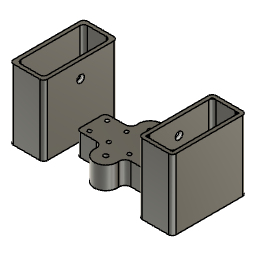
Camera Tilt Mount (Autodesk Fusion 360 design; units mm, degrees)
Autodesk Fusion 360 part; units mm, degrees
sketch "Sketch1" plane through (0, 0, 0) normal (0, 0, 1) x (1, 0, 0)
  circle A0 centre (0, 0) radius 11.25
  line L0 (0, 0) -> (0, 15)
  line L1 (0, 15) -> (0, -15)
  circle A1 centre (0, 15) radius 1.5
  circle A2 centre (0, -15) radius 1.5
  line L2 (0, 0) -> (7.955, -7.955)
  line L3 (0, 0) -> (11.25, 0) construction
  line L4 (0, 0) -> (-7.955, -7.955)
  line L5 (-7.955, -7.955) -> (7.955, -7.955)
  line L6 (-7.955, -7.955) -> (7.955, -7.955)
  line L7 (-7.955, -7.955) -> (-7.955, 7.955)
  line L8 (-7.955, 7.955) -> (7.955, 7.955)
  line L9 (-7.955, 7.955) -> (7.955, 7.955)
  line L10 (0, 0) -> (32.5, 0)
  line L11 (32.5, 0) -> (0, 0)
  line L12 (0, 0) -> (-32.5, 0)
  line L13 (32.5, 0) -> (4.5, 0)
  line L14 (-32.5, 0) -> (-4.5, 0)
  line L15 (-4.5, 0) -> (-22.5, 0)
  line L16 (0, 0) -> (18, 0)
  line L17 (32.5, 0) -> (22.5, 0)
  line L18 (4.5, 0) -> (4.5, 22.5)
  line L19 (4.5, 22.5) -> (22.5, 22.5)
  line L20 (22.5, 22.5) -> (22.5, -22.5)
  line L21 (22.5, -22.5) -> (4.5, -22.5)
  line L22 (4.5, -22.5) -> (4.5, 0)
  line L23 (4.5, 22.5) -> (2, 22.5)
  line L24 (2, 22.5) -> (2, 25)
  line L25 (2, 22.5) -> (2, -25)
  line L26 (2, -25) -> (25, -25)
  line L27 (25, -25) -> (25, 25)
  line L28 (25, 25) -> (2, 25)
  circle A3 centre (0, 15) radius 7.75
  circle A4 centre (0, -15) radius 7.75
  line L29 (-32.5, 0) -> (-4.5, 0)
  line L30 (-4.5, 0) -> (-4.5, 22.5)
  line L31 (-4.5, 22.5) -> (-4.5, -22.5)
  line L32 (-4.5, -22.5) -> (-22.5, -22.5)
  line L33 (-22.5, -22.5) -> (-22.5, 22.5)
  line L34 (-22.5, 22.5) -> (-4.5, 22.5)
  line L35 (-4.5, 22.5) -> (-4.5, 25)
  line L36 (-4.5, 25) -> (-2, 25)
  line L37 (-2, 25) -> (-2, -25)
  line L38 (-2, -25) -> (-25, -25)
  line L39 (-25, -25) -> (-25, 25)
  line L40 (-25, 25) -> (-4.5, 25)
  dimension "d1" = 22.5
  dimension "d2" = 15
  dimension "d3" = 30
  dimension "d4" = 3
  dimension "d5" = 3
  dimension "d6" = 45
  dimension "d7" = 90
  dimension "d10" = 32.5
  dimension "d11" = 32.5
  dimension "d12" = 28
  dimension "d13" = 28
  dimension "d14" = 18
  dimension "d15" = 18
  dimension "d18" = 10
  dimension "d19" = 22.5
  dimension "d20" = 18
  dimension "d21" = 45
  dimension "d22" = 47.5
  dimension "d23" = 23
  dimension "d24" = 15.5
  dimension "d25" = 15.5
  dimension "d26" = 28
  dimension "d27" = 22.5
  dimension "d28" = 45
  dimension "d29" = 18
  constraint coincident A0.centre L0.start
  constraint vertical L0
  constraint parallel L0 L1
  constraint coincident L0.end L1.start
  constraint coincident L1.end A2.centre
  constraint horizontal L3
  constraint coincident A0 L2.end
  constraint coincident A0 L4.end
  constraint horizontal L6
  constraint coincident A0 L7.end
  constraint perpendicular L5 L7
  constraint coincident A0 L8.end
  constraint perpendicular L7 L8
  constraint horizontal L9
  constraint perpendicular L1 L10
  constraint perpendicular L0 L12
  constraint parallel L10 L13
  constraint perpendicular L7 L14
  constraint parallel L12 L15
  constraint parallel L10 L16
  constraint parallel L11 L17
  constraint perpendicular L13 L18
  constraint perpendicular L18 L19
  constraint perpendicular L19 L20
  constraint perpendicular L20 L21
  constraint perpendicular L11 L22
  constraint perpendicular L18 L23
  constraint perpendicular L23 L24
  constraint perpendicular L23 L25
  constraint perpendicular L25 L26
  constraint perpendicular L26 L27
  constraint perpendicular L24 L28
  constraint concentric A1 A3
  constraint concentric A2 A4
  constraint parallel L14 L29
  constraint perpendicular L14 L30
  constraint parallel L30 L31
  constraint perpendicular L31 L32
  constraint perpendicular L32 L33
  constraint perpendicular L30 L34
  constraint perpendicular L34 L35
  constraint perpendicular L35 L36
  constraint perpendicular L36 L37
  constraint perpendicular L37 L38
  constraint perpendicular L38 L39
  constraint perpendicular L35 L40
  measures "d1" diameter of A0
  measures "d2" distance of A0.centre L0.end
  measures "d3" distance of L0.end L1.end
  measures "d4" diameter of A1
  measures "d5" diameter of A2
  measures "d6" angle of L2 L3
  measures "d7" angle of L2 L4
  measures "d10" distance of A0.centre L10.end
  measures "d11" distance of A0.centre L12.end
  measures "d12" distance of L10.end L13.end
  measures "d13" distance of L12.end L14.end
  measures "d14" distance of L14.end L15.end
  measures "d15" distance of A0.centre L16.end
  measures "d18" distance of L10.end L17.end
  measures "d19" distance of L13.end L18.end
  measures "d20" distance of L18.end L19.end
  measures "d21" distance of L19.end L20.end
  measures "d22" distance of L23.end L25.end
  measures "d23" distance of L25.end L26.end
  measures "d24" diameter of A3
  measures "d25" diameter of A4
  measures "d26" distance of L12.end L14.end
  measures "d27" distance of L14.end L30.end
  measures "d28" distance of L30.end L31.end
  measures "d29" distance of L31.end L32.end
extrude "Extrude1" add sketch "Sketch1" along normal blind 50 contours L2 L10 L11 L16 L22 L25 | L8 L9 L10 L11 L16 L18 L25 A3 | L8 L9 L18 A3 | L2 L5 L6 L22 L25 A4 | L5 L6 L22 A4 | L10 L11 L13 L17 L19 L20 L23 L24 L27 L28 | L10 L11 L13 L17 L20 L21 L22 L25 L26 L27 A4 | A0 L8 L9 L18 L25 A3 | A0 L18 L25 A3 | L8 L9 L25 A3 | A0 L22 L25 A4 | A0 L5 L6 L22 L25 A4 | L5 L6 L25 A4 | L18 L23 L25 A3 | L4 L5 L6 A4 L31 L37 | L4 L12 L31 L37 | L8 L9 L12 A3 L30 L31 L37 | L8 L9 A3 L37 | L5 L6 A4 L37 | A0 L8 L9 A3 L30 L31 L37 | A0 A3 L30 L31 L37 | A3 L30 L31 L35 L36 L37 | A0 A4 L31 L37 | A0 L5 L6 A4 L31 L37 | L12 L14 A4 L29 L31 L32 L33 L37 L38 L39 | L8 L9 A3 L30 L31 | L5 L6 A4 L31 | L12 L14 L29 L33 L34 L35 L39 L40 makes body 1 at (-2, 8.3333, 16.6667) makes body 2 at (2, 8.3333, 16.6667)
extrude "Extrude2" add sketch "Sketch1" along normal blind 2.5 separate body contours A0 L8 L9 L10 L11 L13 L16 L18 | A0 L10 L11 L13 L16 L20 L21 L22 A4 | A0 L2 L10 L11 L13 L16 L22 | A0 L10 L11 L13 L16 L18 L19 L20 A3 | A0 L8 L9 L18 A3 | L2 L5 L6 L22 | A0 L5 L6 L22 A4 | A0 L18 A3 | A0 L18 A3 | A0 L22 A4 | A0 L22 A4 | L4 L5 L6 L31 | L4 L7 L12 L14 L15 L29 L31 | L7 L8 L9 L12 L14 L15 L29 L30 L31 | A0 L12 L14 L15 A4 L29 L31 L32 L33 | A0 L5 L6 A4 L31 | A0 L7 L12 L14 L15 L29 | A0 L7 L12 L14 L15 L29 | A0 L8 L9 A3 L30 L31 | A0 A3 L30 L31 | A0 A3 L30 L31 | A0 L12 L14 L15 A3 L29 L30 L31 L33 L34 | A0 A4 L31 | A0 A4 L31 makes body 3 at (-10.5, -7.5, 0) makes body 4 at (16.5, -7.5, 0)
extrude "Extrude4" add sketch "Sketch1" against normal blind 10 separate body contours A0 L8 L9 L10 L11 L13 L16 L18 | A0 L2 L10 L11 L13 L16 L22 | A0 L8 L9 L18 A3 | L2 L5 L6 L22 | A0 L5 L6 L22 A4 | L2 L10 L11 L16 L22 L25 | L8 L9 L10 L11 L16 L18 L25 A3 | A0 L18 A3 | A0 L18 A3 | L8 L9 L18 A3 | A0 L22 A4 | A0 L22 A4 | L2 L5 L6 L22 L25 A4 | L5 L6 L22 A4 | L2 L10 L11 L16 L25 | L0 L1 L10 L11 L16 L25 A3 | A0 L8 L9 L18 L25 A3 | A0 L18 L25 A3 | L8 L9 L25 A3 | A0 L22 L25 A4 | A0 L5 L6 L22 L25 A4 | L1 L2 L25 A4 | L5 L6 L25 A4 | L0 L1 L12 A3 L37 | L1 L4 A4 L37 | L4 L12 L37 | L0 L1 L8 L9 L25 A3 | A0 L0 L1 L8 L9 L25 | A0 L25 A3 L37 | A0 L25 A4 L37 | A0 L1 L5 L6 L25 | L1 L5 L6 L25 A4 | L0 L1 L8 L9 A3 L37 | L1 L5 L6 A4 L37 | L4 L5 L6 A4 L31 L37 | L4 L12 L31 L37 | L8 L9 L12 A3 L30 L31 L37 | A0 L0 L1 L8 L9 L37 | A0 L1 L5 L6 L37 | L8 L9 A3 L37 | L5 L6 A4 L37 | L4 L5 L6 L31 | L4 L7 L12 L14 L15 L29 L31 | L7 L8 L9 L12 L14 L15 L29 L30 L31 | A0 L8 L9 A3 L30 L31 L37 | A0 A3 L30 L31 L37 | A0 A4 L31 L37 | A0 L5 L6 A4 L31 L37 | L8 L9 A3 L30 L31 | L5 L6 A4 L31 | A0 L5 L6 A4 L31 | A0 L7 L12 L14 L15 L29 | A0 L7 L12 L14 L15 L29 | A0 L8 L9 A3 L30 L31 | A0 A3 L30 L31 | A0 A3 L30 L31 | A0 A4 L31 | A0 A4 L31 makes body 5
extrude "Extrude5" add sketch "Sketch1" along normal blind 2.5 contours A0 L8 L9 L10 L11 L13 L16 L18 | A0 L10 L11 L13 L16 L20 L21 L22 A4 | A0 L2 L10 L11 L13 L16 L22 | A0 L10 L11 L13 L16 L18 L19 L20 A3 | A0 L8 L9 L18 A3 | L2 L5 L6 L22 | A0 L5 L6 L22 A4 | A0 L18 A3 | A0 L18 A3 | A0 L22 A4 | A0 L22 A4 | L4 L5 L6 L31 | L4 L7 L12 L14 L15 L29 L31 | L7 L8 L9 L12 L14 L15 L29 L30 L31 | A0 L12 L14 L15 A4 L29 L31 L32 L33 | A0 L5 L6 A4 L31 | A0 L7 L12 L14 L15 L29 | A0 L7 L12 L14 L15 L29 | A0 L8 L9 A3 L30 L31 | A0 A3 L30 L31 | A0 A3 L30 L31 | A0 L12 L14 L15 A3 L29 L30 L31 L33 L34 | A0 A4 L31 | A0 A4 L31 bodies 5
extrude "Extrude6" cut sketch "Sketch1" along normal blind 1 contours A0 L8 L9 L10 L11 L13 L16 L18 | A0 L10 L11 L13 L16 L20 L21 L22 A4 | A0 L2 L10 L11 L13 L16 L22 | A0 L10 L11 L13 L16 L18 L19 L20 A3 | A0 L8 L9 L18 A3 | L2 L5 L6 L22 | A0 L5 L6 L22 A4 | A0 L18 A3 | A0 L18 A3 | A0 L22 A4 | A0 L22 A4 | L4 L5 L6 L31 | L4 L7 L12 L14 L15 L29 L31 | L7 L8 L9 L12 L14 L15 L29 L30 L31 | A0 L12 L14 L15 A4 L29 L31 L32 L33 | A0 L5 L6 A4 L31 | A0 L7 L12 L14 L15 L29 | A0 L7 L12 L14 L15 L29 | A0 L8 L9 A3 L30 L31 | A0 A3 L30 L31 | A0 A3 L30 L31 | A0 L12 L14 L15 A3 L29 L30 L31 L33 L34 | A0 A4 L31 | A0 A4 L31 bodies 5 makes body 6 at (-10.5, -7.5, 1) makes body 7 at (2.8306, -3.9262, -10)
extrude "Extrude7" add sketch "Sketch1" along normal blind 50 contours L2 L10 L11 L16 L22 L25 | L8 L9 L10 L11 L16 L18 L25 A3 | L8 L9 L18 A3 | L2 L5 L6 L22 L25 A4 | L5 L6 L22 A4 | L10 L11 L13 L17 L19 L20 L23 L24 L27 L28 | L10 L11 L13 L17 L20 L21 L22 L25 L26 L27 A4 | A0 L8 L9 L18 L25 A3 | A0 L18 L25 A3 | L8 L9 L25 A3 | A0 L22 L25 A4 | A0 L5 L6 L22 L25 A4 | L5 L6 L25 A4 | L18 L23 L25 A3 | L4 L5 L6 A4 L31 L37 | L4 L12 L31 L37 | L8 L9 L12 A3 L30 L31 L37 | L8 L9 A3 L37 | L5 L6 A4 L37 | A0 L8 L9 A3 L30 L31 L37 | A0 A3 L30 L31 L37 | A3 L30 L31 L35 L36 L37 | A0 A4 L31 L37 | A0 L5 L6 A4 L31 L37 | L12 L14 A4 L29 L31 L32 L33 L37 L38 L39 | L8 L9 A3 L30 L31 | L5 L6 A4 L31 | L12 L14 L29 L33 L34 L35 L39 L40 bodies 5 6 7
extrude "Extrude8" cut sketch "Sketch1" along normal blind 1 contours L2 L10 L11 L16 L22 L25 | L8 L9 L10 L11 L16 L18 L25 A3 | L8 L9 L18 A3 | L2 L5 L6 L22 L25 A4 | L5 L6 L22 A4 | L10 L11 L13 L17 L19 L20 L23 L24 L27 L28 | L10 L11 L13 L17 L20 L21 L22 L25 L26 L27 A4 | A0 L8 L9 L18 L25 A3 | A0 L18 L25 A3 | L8 L9 L25 A3 | A0 L22 L25 A4 | A0 L5 L6 L22 L25 A4 | L5 L6 L25 A4 | L18 L23 L25 A3 | L4 L5 L6 A4 L31 L37 | L4 L12 L31 L37 | L8 L9 L12 A3 L30 L31 L37 | L8 L9 A3 L37 | L5 L6 A4 L37 | A0 L8 L9 A3 L30 L31 L37 | A0 A3 L30 L31 L37 | A3 L30 L31 L35 L36 L37 | A0 A4 L31 L37 | A0 L5 L6 A4 L31 L37 | L12 L14 A4 L29 L31 L32 L33 L37 L38 L39 | L8 L9 A3 L30 L31 | L5 L6 A4 L31 | L12 L14 L29 L33 L34 L35 L39 L40 bodies 5 makes body 8 at (2, 8.3333, 17.3333) makes body 9 at (-2, 8.3333, 17.3333)
extrude "Extrude9" add 2 faces at (24.1667, 7.5, 50) (-24.1667, 7.5, 50) along direction (0, 0, 1) blind 1 on bodies 8 9 bodies 8 9
sketch "Sketch2" plane through (0, 0, -10) normal (0, 0, -1) x (1, 0, 0)
  circle A0 centre (0, 15) radius 1.5
  circle A1 centre (0, -15) radius 1.5
  arc A2 (5.67, 9.7167) -> (-5.67, 9.7167) centre (0, 15) ccw
  arc A3 (-5.67, 9.7167) -> (-5.67, -9.7167) centre (0, 0) ccw
  arc A4 (-5.67, -9.7167) -> (5.67, -9.7167) centre (0, -15) ccw
  arc A5 (5.67, -9.7167) -> (5.67, 9.7167) centre (0, 0) ccw
  line L0 (0, 0) -> (15, 0)
  line L1 (15, 0) -> (-15, 0)
  line L2 (-5.67, 9.7167) -> (-25, 9.7167)
  line L3 (5.67, 9.7167) -> (25, 9.7167)
  line L4 (5.67, -9.7167) -> (25, -9.7167)
  line L5 (-5.67, -9.7167) -> (-25, -9.7167)
  line L6 (-25, -9.7167) -> (-25, 9.7167)
  line L7 (25, 9.7167) -> (25, -9.7167)
  line L8 (25, 9.7167) -> (22.5, 9.7167)
  line L9 (22.5, 9.7167) -> (20, 9.7167)
  line L10 (20, 9.7167) -> (20, -9.7167)
  line L11 (-25, 9.7167) -> (-20, 9.7167)
  line L12 (-20, 9.7167) -> (-20, -9.7167)
  line L13 (-20, 0) -> (-20, -6)
  line L14 (-20, -6) -> (-20, 6)
  line L15 (-20, 6) -> (20, 6)
  line L16 (20, 6) -> (20, -6)
  line L17 (-20, 6) -> (-25, 6)
  line L18 (-2, 6) -> (-7, 6)
  line L19 (-7, 6) -> (-7, -6)
  line L20 (2, 6) -> (7, 6)
  line L21 (7, 6) -> (7, -6)
  dimension "d50" = 2.5
  constraint coincident A3.centre A5.centre
  constraint horizontal L0
  constraint parallel L0 L1
  constraint coincident A2.end A3.start
  constraint parallel L1 L2
  constraint coincident A2.start A5.end
  constraint horizontal L3
  constraint coincident A4.end A5.start
  constraint horizontal L4
  constraint coincident A3.end A4.start
  constraint horizontal L5
  constraint perpendicular L4 L7
  constraint perpendicular L7 L8
  constraint coincident L3 L9.end
  constraint coincident L4 L10.end
  constraint perpendicular L4 L10
  constraint coincident L2 L11.end
  constraint coincident L5 L12.end
  constraint perpendicular L5 L12
  constraint midpoint L12 L13.start
  constraint coincident L12 L13.end
  constraint perpendicular L5 L13
  constraint coincident L12 L14.end
  constraint perpendicular L12 L15
  constraint coincident L10 L16.end
  constraint perpendicular L15 L16
  constraint coincident L6 L17.end
  constraint perpendicular L6 L17
  constraint coincident L15 L18.start
  constraint coincident L15 L18.end
  constraint perpendicular L12 L18
  constraint perpendicular L1 L19
  constraint coincident L15 L20.start
  constraint coincident L15 L20.end
  constraint perpendicular L1 L21
  measures "d50" distance of L3.end L8.end
extrude "Extrude11" add sketch "Sketch2" against normal blind 10 contours A5 L3 L10 L15 | A3 L2 L12 L15 | A5 L4 L10 L15 L16 | L3 L4 L7 L8 L9 L10 L16 | A3 L5 L12 L13 L14 L15 bodies 5
extrude "Extrude10" add sketch "Sketch2" against normal blind 10 contours A5 L3 L10 L15 | A3 L2 L12 L15 | A5 L4 L10 L15 L16 | L3 L4 L7 L8 L9 L10 L16 | A3 L5 L12 L13 L14 L15 | L2 L6 L11 L12 L17 | L5 L6 L12 L13 L14 L17 bodies 5
hole "Hole1" at (-20, -6, -10) direction (0, 0, 1) diameter 2.529 depth 20 tip angle 118 bodies 3 5 9
thread "Thread1" "ISO Metric profile 3.0 M3x0.5 6H" major diameter 3.086 minor diameter 2.529 pitch 0.5 angle 60 resizes the face on face at (-19.937, -4.7371, -6.6667) on face at (-19.937, -4.7371, 1.5) on face at (-19.937, -4.7371, 0.8333) on bodies 3 5 9
hole "Hole2" at (20, -6, -10) direction (0, 0, 1) diameter 2.529 depth 20 tip angle 118 bodies 4 5 8
thread "Thread2" "ISO Metric profile 3.0 M3x0.5 6H" major diameter 3.086 minor diameter 2.529 pitch 0.5 angle 60 resizes the face on face at (20.063, -4.7371, 0.8333) on face at (20.063, -4.7371, 1.5) on face at (20.063, -4.7371, -6.6667) on bodies 4 5 8
hole "Hole3" at (-20, 6, -10) direction (0, 0, 1) diameter 2.529 depth 20 tip angle 118 bodies 3 5 9
thread "Thread3" "ISO Metric profile 3.0 M3x0.5 6H" major diameter 3.086 minor diameter 2.529 pitch 0.5 angle 60 resizes the face on face at (-19.937, 7.2629, 0.8333) on face at (-19.937, 7.2629, -6.6667) on face at (-19.937, 7.2629, 1.5) on bodies 3 5 9
hole "Hole4" at (20, 6, -10) direction (0, 0, 1) diameter 2.529 depth 20 tip angle 118 bodies 4 5 8
thread "Thread4" "ISO Metric profile 3.0 M3x0.5 6H" major diameter 3.086 minor diameter 2.529 pitch 0.5 angle 60 resizes the face on face at (20.063, 7.2629, 1.5) on face at (20.063, 7.2629, -6.6667) on face at (20.063, 7.2629, 0.8333) on bodies 4 5 8
hole "Hole5" at (-7, -6, -10) direction (0, 0, 1) diameter 2.529 depth 20 tip angle 118 bodies 3 5 9
thread "Thread5" "ISO Metric profile 3.0 M3x0.5 6H"
hole "Hole6" at (-7, 6, -10) direction (0, 0, 1) diameter 2.529 depth 20 tip angle 118 bodies 3 5 9
thread "Thread6" "ISO Metric profile 3.0 M3x0.5 6H"
hole "Hole7" at (7, -6, -10) direction (0, 0, 1) diameter 2.529 depth 20 tip angle 118 bodies 4 5 8
thread "Thread7" "ISO Metric profile 3.0 M3x0.5 6H"
hole "Hole8" at (7, 6, -10) direction (0, 0, 1) diameter 2.529 depth 20 tip angle 118 bodies 4 5 8
thread "Thread8" "ISO Metric profile 3.0 M3x0.5 6H"
extrude "Extrude12" cut 4 faces at (-24.1667, 7.5, 0) (-11.5708, 17.3483, 0) (24.1667, 7.5, 0) (11.5708, -17.3483, 0) along direction (0, 0, 1) blind 1 on bodies 1 2 3 4 bodies 1 2 3 4
move_body "Move1" bodies 1 3 9 to x (1, 0, 0) y (0, 1, 0) z (0, 0, 1) at (-30, 0, 0)
move_body "Move2" bodies 2 4 8 to x (1, 0, 0) y (0, 1, 0) z (0, 0, 1) at (30, 0, 0)
sketch "Sketch3" plane through (-32, 0, 0) normal (1, 0, 0) x (0, 1, 0)
  line L0 (-25, 1) -> (25, 1)
  line L1 (25, 1) -> (25, 51)
  line L2 (25, 51) -> (-25, 51)
  line L3 (-25, 51) -> (-25, 1)
  line L4 (-25, 1) -> (25, 51)
  line L5 (25, 1) -> (-25, 51)
  line L6 (0, 26) -> (0, 1)
  line L7 (0, 1) -> (0, 3.5)
  line L8 (0, 3.5) -> (0, 37.5)
  dimension "d87" = 2.5
  dimension "d88" = 34
  constraint coincident L0.start L3.end
  constraint coincident L1.end L2.start
  constraint coincident L0.end L1.start
  constraint coincident L2.end L3.start
  constraint midpoint L5 L6.start
  constraint midpoint L0 L6.end
  constraint perpendicular L0 L7
  constraint parallel L6 L8
  measures "d87" distance of L6.end L7.end
  measures "d88" distance of L7.end L8.end
hole "Hole9" at (-32, 0, 37.5) direction (-1, 0, 0) diameter 5.035 depth 5 tip angle 118 bodies 9 1
thread "Thread9" "ISO Metric profile 6.0 M6x1 6H"
extrude "Extrude13" add 1 faces at (41.5708, 17.3483, 2.5) along direction (0, 0, 1) blind 1 on bodies 8 bodies 8 4
extrude "Extrude14" cut 1 faces at (54.1667, 7.5, 51) along direction (0, 0, -1) blind 2.5 on bodies 8 bodies 8
extrude "Extrude15" add 1 faces at (-41.5708, 17.3483, 2.5) along direction (0, 0, 1) blind 1 on bodies 9 bodies 9 1
extrude "Extrude16" cut 1 faces at (-54.1667, 7.5, 51) along direction (0, 0, -1) blind 2.5 on bodies 9 bodies 9
sketch "Sketch4" plane through (32, 0, 0) normal (-1, 0, 0) x (0, -1, 0)
  line L0 (25, 48.5) -> (-25, 48.5)
  line L1 (-25, 48.5) -> (-25, 1)
  line L2 (-25, 1) -> (25, 1)
  line L3 (25, 1) -> (25, 48.5)
  line L4 (0, 1) -> (0, 3.5)
  line L5 (0, 3.5) -> (0, 37.5)
  dimension "d92" = 2.5
  dimension "d93" = 34
  constraint midpoint L2 L4.start
  constraint perpendicular L2 L4
  constraint parallel L4 L5
  measures "d92" distance of L4.start L4.end
  measures "d93" distance of L4.end L5.end
hole "Hole10" at (32, 0, 37.5) direction (1, 0, 0) diameter 5.035 depth 5 tip angle 118 bodies 8
thread "Thread10" "ISO Metric profile 6.0 M6x1 6H"
extrude "Extrude17" cut 1 faces at (54.1667, 7.5, 50) along direction (0, 0, -1) blind 1.5 on bodies 2 bodies 2
fillet "Fillet1" radius 4 1 edges at (-5.67, -9.7167, -5) on bodies 5
fillet "Fillet2" radius 4 1 edges at (5.67, -9.7167, -5) on bodies 5
fillet "Fillet3" radius 4 1 edges at (5.67, 9.7167, -5) on bodies 5
fillet "Fillet4" radius 4 1 edges at (-5.67, 9.7167, -5) on bodies 5
sketch "Sketch5" plane through (32, 0, 0) normal (-1, 0, 0) x (0, -1, 0)
  line L0 (25, 48.5) -> (-25, 48.5)
  line L1 (-25, 48.5) -> (-25, 1)
  line L2 (-25, 1) -> (25, 1)
  line L3 (25, 1) -> (25, 48.5)
  line L4 (0, 40) -> (0, 35)
  line L5 (0, 35) -> (0, 37.5)
  dimension "d107" = 2.5
  constraint vertical L4
  constraint parallel L4 L5
  measures "d107" distance of L4.end L5.end
hole "Hole11" at (32, 0, 37.5) direction (1, 0, 0) diameter 5.035 depth 5 tip angle 118 bodies 2
thread "Thread11" "ISO Metric profile 6.0 M6x1 6H"
fillet "Fillet5" radius 2.5 1 edges at (52.5, -22.5, 26) on bodies 8
fillet "Fillet6" radius 2.5 1 edges at (34.5, -22.5, 24.75) on bodies 2
fillet "Fillet7" radius 2.5 1 edges at (34.5, 22.5, 26) on bodies 8
fillet "Fillet8" radius 2.5 1 edges at (52.5, 22.5, 24.75) on bodies 2
fillet "Fillet9" radius 2.5 1 edges at (32, 25, 24.75) on bodies 8
fillet "Fillet10" radius 2.5 1 edges at (32, 25, 24.75) on bodies 2
fillet "Fillet11" radius 2.5 1 edges at (55, 25, 24.75) on bodies 8
fillet "Fillet12" radius 2.5 1 edges at (55, 25, 24.75) on bodies 2
fillet "Fillet13" radius 2.5 6 edges at (32, -25, 24.75) (55, -25, 24.75) (-55, -25, 24.75) (-32, -25, 24.75) (-55, 25, 24.75) (-32, 25, 24.75) on bodies 8 9
fillet "Fillet14" radius 2.5 4 edges at (-34.5, -22.5, 26) (-52.5, -22.5, 26) (-34.5, 22.5, 26) (-52.5, 22.5, 26) on bodies 9
fillet "Fillet15" radius 2.5 1 edges at (55, -25, 24.75) on bodies 2
fillet "Fillet16" radius 2.5 1 edges at (32, -25, 24.75) on bodies 2
fillet "Fillet17" radius 2.5 4 edges at (-25, -9.7167, -5) (25, -9.7167, -5) (25, 9.7167, -5) (-25, 9.7167, -5) on bodies 5
move_body "Move3" bodies 2 3 8 9 to x (1, 0, 0) y (0, 1, 0) z (0, 0, 1) at (0, 0, -11)
sketch "Sketch6" plane through (0, 0, 0) normal (0, 1, 0) x (1, 0, 0)
extrude "Extrude18" add 1 faces at (-2.0038, 1.7372, 0) along direction (0, 0, 1) blind 5 on bodies 5 bodies 5
